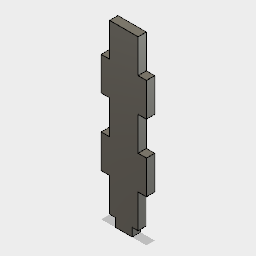
servo_guide2 v2 (Autodesk Fusion 360 design; units mm, degrees)
Autodesk Fusion 360 part; units mm, degrees
sketch "スケッチ1" plane through (0, 0, 0) normal (0, 0, 1) x (1, 0, 0)
  line L0 (35.16, -63.4696) -> (35.16, -53.4695)
  line L1 (35.16, -53.4695) -> (32.66, -53.4695)
  line L2 (32.66, -53.4695) -> (32.66, -43.4694)
  line L3 (32.66, -43.4694) -> (35.16, -43.4694)
  line L4 (35.16, -43.4694) -> (35.16, -33.4693)
  line L5 (35.16, -33.4693) -> (32.66, -33.4693)
  line L6 (32.66, -33.4693) -> (32.66, -23.4692)
  line L7 (32.66, -23.4692) -> (35.16, -23.4692)
  line L8 (35.16, -23.4692) -> (35.16, -13.4691)
  line L9 (35.16, -13.4691) -> (43.6602, -13.4691)
  line L10 (43.6602, -13.4691) -> (43.6602, -23.4692)
  line L11 (43.6602, -23.4692) -> (46.1602, -23.4692)
  line L12 (46.1602, -23.4692) -> (46.1602, -33.4693)
  line L13 (46.1602, -33.4693) -> (43.6602, -33.4693)
  line L14 (43.6602, -33.4693) -> (43.6602, -43.4694)
  line L15 (43.6602, -43.4694) -> (46.1602, -43.4694)
  line L16 (46.1602, -43.4694) -> (46.1602, -53.4695)
  line L17 (46.1602, -53.4695) -> (43.6602, -53.4695)
  spline S0 degree 3 poles (43.6602, -53.4695) (43.6602, -53.4695) (43.6602, -63.4696) (43.6601, -63.4696) knots 18 18 18 18 19 19 19 19
  line L18 (43.6601, -63.4696) -> (41.9101, -63.4696)
  line L19 (41.9101, -63.4696) -> (41.9101, -65.9695)
  line L20 (41.9101, -65.9695) -> (36.9101, -65.9695)
  line L21 (36.9101, -65.9695) -> (36.9101, -63.4696)
  line L22 (36.9101, -63.4696) -> (35.16, -63.4696)
extrude "押し出し1" add sketch "スケッチ1" along normal blind 2.5
